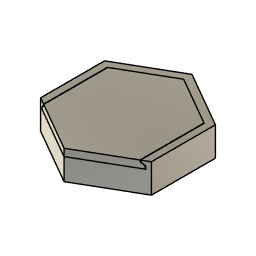
HexStore2 (Autodesk Fusion 360 design; units mm, degrees)
Autodesk Fusion 360 part; units mm, degrees
sketch "Sketch1" plane through (0, 0, 0) normal (0, 0, 1) x (1, 0, 0)
  line L0 (0, -46.188) -> (40, -23.094)
  line L1 (40, -23.094) -> (40, 23.094)
  line L2 (40, 23.094) -> (0, 46.188)
  line L3 (0, 46.188) -> (-40, 23.094)
  line L4 (-40, 23.094) -> (-40, -23.094)
  line L5 (-40, -23.094) -> (0, -46.188)
  line L6 (-46, 26.5581) -> (-46, -26.5581)
  line L7 (-46, -26.5581) -> (0, -53.1162)
  line L8 (0, -53.1162) -> (46, -26.5581)
  line L9 (46, -26.5581) -> (46, 26.5581)
  line L10 (46, 26.5581) -> (0, 53.1162)
  line L11 (0, 53.1162) -> (-46, 26.5581)
  dimension "d1" = 40
  dimension "d2" = 6
  constraint vertical L1
  measures "d1" distance of origin L5
extrude "Extrude1" add sketch "Sketch1" along normal blind 2 contours L0 L1 L2 L3 L4 L5 | L6 L7 L8 L9 L10 L11 makes body 1 in component "Case"
extrude "Extrude2" add sketch "Sketch1" along normal blind 24 bodies 1 in component "Case"
ref_plane "WorkPlane1" through (-46, -26.5581, 0) normal (0, -1, 0) x (1, 0, 0)
sketch "Sketch2" plane through (0, -26.5581, 0) normal (0, -1, 0) x (-1, 0, 0)
  line L0 (0, -24) -> (40, -24)
  line L1 (40, -24) -> (0, -24)
  line L2 (0, -24) -> (-40, -24)
  line L3 (-40, -24) -> (0, -24)
  line L4 (0, -24) -> (46, -24)
  line L5 (46, -24) -> (0, -24)
  line L6 (0, -24) -> (-46, -24)
  line L7 (-46, -24) -> (0, -24)
  line L8 (46, -24) -> (43, -24)
  line L9 (43, -24) -> (43, -18)
  line L10 (43, -18) -> (46, -18)
  line L11 (46, -18) -> (46, -24)
  line L12 (43, -24) -> (40, -24)
  line L13 (40, -24) -> (40, -18)
  line L14 (40, -18) -> (43, -18)
  line L15 (43, -18) -> (43, -24)
  line L16 (40.19, -24) -> (40.19, -23)
  line L17 (40.19, -23) -> (43, -20.19)
  line L18 (42.81, -18) -> (42.81, -20.1113)
  line L19 (42.81, -20.1113) -> (40, -22.9213)
  line L20 (0, 0) -> (0, -24)
  line L21 (-43, -24) -> (-40, -24)
  line L22 (-40, -18) -> (-43, -18)
  line L23 (-43, -18) -> (-43, -24)
  line L24 (-40, -24) -> (-40, -18)
  line L25 (-43, -24) -> (-43, -18)
  line L26 (-46, -18) -> (-46, -24)
  line L27 (-46, -24) -> (-43, -24)
  line L28 (-43, -18) -> (-46, -18)
  line L29 (-42.81, -18) -> (-42.81, -20.1113)
  line L30 (-42.81, -20.1113) -> (-40, -22.9213)
  line L31 (-40.19, -23) -> (-43, -20.19)
  line L32 (-40.19, -24) -> (-40.19, -23)
  line L33 (40, -18) -> (-40, -18)
  dimension "d7" = 3
  dimension "d8" = 6
  dimension "d9" = 3
  dimension "d10" = 6
  dimension "d11" = 45
  dimension "d12" = 0.19
  dimension "d13" = 0.19
  dimension "d14" = 0.19
  dimension "d15" = 1
  constraint horizontal L8
  constraint vertical L9
  constraint horizontal L10
  constraint vertical L11
  constraint coincident L4.end L5.start
  constraint horizontal L12
  constraint vertical L13
  constraint horizontal L14
  constraint vertical L15
  constraint coincident L12 L16.start
  constraint perpendicular L4 L16
  constraint coincident L15 L17.end
  constraint coincident L14 L18.start
  constraint perpendicular L14 L18
  constraint coincident L13 L19.end
  constraint parallel L17 L19
  constraint symmetric L4.end L20 L6.end
  constraint symmetric L8.end L20 L21.start
  constraint symmetric L9.end L20 L22.end
  constraint symmetric L10.end L20 L26.start
  constraint symmetric L0.end L20 L2.end
  constraint symmetric L13.end L20 L22.start
  constraint symmetric L16.start L20 L32.start
  constraint symmetric L16.end L20 L31.start
  constraint symmetric L17.end L20 L31.end
  constraint symmetric L18.start L20 L29.start
  constraint symmetric L18.end L20 L29.end
  constraint symmetric L19.end L20 L30.end
  measures "d7" distance of L4.end L8.end
  measures "d8" distance of L4.end L10.end
  measures "d9" distance of L8.end L0.end
  measures "d10" distance of L8.end L9.end
  measures "d11" angle of L9 L17
  measures "d12" distance of L15 L18
  measures "d13" distance of L17 L19
  measures "d14" distance of L13 L16
  measures "d15" distance of L16.start L16.end
extrude "Extrude3" cut sketch "Sketch2" along normal up to surface (-49.6521 mm away) and the other way up to surface (-26.5581 mm away) contours L0 L1 L4 L5 L13 L20 L33 | L2 L3 L6 L7 L20 L24 L33 | L4 L5 L9 L12 L13 L14 L15 L16 L17 L18 L19 | L6 L7 L21 L22 L23 L24 L25 L29 L30 L31 L32 | L13 L14 L18 L19 | L22 L24 L29 L30 bodies 1 in component "Case"
extrude "Extrude1'" add sketch "Sketch1" along normal blind 6 from surface at 18 separate body contours L0 L1 L2 L3 L4 L5 | L6 L7 L8 L9 L10 L11 makes body 2 in component "Lid"
extrude "Extrude2'" cut sketch "Sketch2" along normal up to surface (-79.6743 mm away) and the other way up to surface (-26.5581 mm away) contours L4 L5 L9 L12 L13 L14 L15 L16 L17 L18 L19 | L6 L7 L21 L22 L23 L24 L25 L29 L30 L31 L32 | L4 L5 L9 L12 L15 L16 L17 | L6 L7 L21 L23 L25 L31 L32 | L4 L5 L8 L9 L10 L11 L15 | L6 L7 L23 L25 L26 L27 L28 bodies 2 in component "Lid"
sketch "Sketch1 (2)" plane through (0, 0, 24) normal (0, 0, 1) x (-1, 0, 0) in component "Lid"
  line L0 (-40, 30.0222) -> (-40, -30.0222)
  line L1 (-40, -30.0222) -> (0, -53.1162)
  line L2 (0, -53.1162) -> (40, -30.0222)
  line L3 (40, -30.0222) -> (40, 30.0222)
  line L4 (40, 30.0222) -> (0, 53.1162)
  line L5 (0, 53.1162) -> (-40, 30.0222)
  line L6 (40, -23.094) -> (-40, -23.094)
  line L7 (-40.19, -23.094) -> (-40.19, 29.9125)
  line L8 (-40.19, 29.9125) -> (-46, 26.5581)
  line L9 (-46, 26.5581) -> (-46, -26.5581)
  line L10 (-46, -26.5581) -> (0, -53.1162)
  line L11 (0, -53.1162) -> (46, -26.5581)
  line L12 (46, -26.5581) -> (46, 26.5581)
  line L13 (46, 26.5581) -> (40.19, 29.9125)
  line L14 (40.19, 29.9125) -> (40.19, -23.094)
  line L15 (40.19, -23.094) -> (40, -23.094)
  line L16 (40, -23.094) -> (0, -46.188)
  line L17 (0, -46.188) -> (-40, -23.094)
  line L18 (-40, -23.094) -> (-40.19, -23.094)
  line L19 (-40.19, -23.094) -> (-46, -23.094)
  line L20 (40, -23.094) -> (46, -23.094)
  point P0 (40, -23.094)
  point P1 (-40, -23.094)
  constraint coincident P0 L6.start
  constraint coincident P1 L6.end
  constraint coincident L7.start L18.end
  constraint coincident L9 L19.end
  constraint perpendicular L9 L19
  constraint coincident L12 L20.end
  constraint perpendicular L12 L20
extrude "Extrude3'" cut sketch "Sketch1 (2)" against normal blind 6 contours L0 L1 L2 L3 L10 L11 L16 L17 | L0 L9 L10 L18 L19 | L3 L11 L12 L15 L20 bodies 2 in component "Lid"
sketch "Sketch1 (3)" plane through (0, 0, 18) normal (0, 0, 1) x (-1, 0, 0) in component "Case"
  line L0 (0, 53.1162) -> (-43, 28.2902)
  line L1 (-43, 28.2902) -> (-43, -23.094)
  line L2 (-43, -23.094) -> (-40, -23.094)
  line L3 (-40, -23.094) -> (-40, 23.094)
  line L4 (-40, 23.094) -> (0, 46.188)
  line L5 (0, 46.188) -> (40, 23.094)
  line L6 (40, 23.094) -> (40, -23.094)
  line L7 (40, -23.094) -> (43, -23.094)
  line L8 (43, -23.094) -> (43, 28.2902)
  line L9 (43, 28.2902) -> (0, 53.1162)
  circle A0 centre (-43, -17.094) radius 0.6
  circle A1 centre (43, -17.094) radius 0.6
  dimension "d30" = 1.2
  dimension "d31" = 1.2
  dimension "d32" = 6
  dimension "d33" = 6
  constraint coincident L1 A0.centre
  constraint coincident L8 A1.centre
  measures "d30" diameter of A0
  measures "d31" diameter of A1
  measures "d32" distance of L7.end A1.centre
  measures "d33" distance of L1.end A0.centre
extrude "Extrude4" add sketch "Sketch1 (3)" along normal blind 6 contours L1 A0 | L8 A1 picked at (-42.8071, -16.9197) picked at (42.805, -17.1385) bodies 1 in component "Case"
sketch "Sketch2 (2)" plane through (0, 0, 18) normal (0, 0, -1) x (1, 0, 0) in component "Lid"
  line L0 (40, -23.094) -> (42.81, -23.094)
  line L1 (42.81, -23.094) -> (42.81, 28.3999)
  line L2 (42.81, 28.3999) -> (0, 53.1162)
  line L3 (0, 53.1162) -> (-42.81, 28.3999)
  line L4 (-42.81, 28.3999) -> (-42.81, -23.094)
  line L5 (-42.81, -23.094) -> (-40, -23.094)
  line L6 (-40, -23.094) -> (0, -46.188)
  line L7 (0, -46.188) -> (40, -23.094)
  circle A0 centre (42.81, -17.094) radius 0.6
  circle A1 centre (-42.81, -17.094) radius 0.6
  dimension "d36" = 1.2
  dimension "d37" = 1.2
  dimension "d38" = 6
  dimension "d39" = 6
  constraint coincident L1 A0.centre
  constraint coincident L4 A1.centre
  measures "d36" diameter of A0
  measures "d37" diameter of A1
  measures "d38" distance of L0.end A0.centre
  measures "d39" distance of L4.end A1.centre
extrude "Extrude4'" cut sketch "Sketch2 (2)" against normal blind 6 contours L1 A0 | L4 A1 picked at (42.6536, -17.2187) picked at (-42.6019, -16.963) bodies 2 in component "Lid"
fillet "Fillet1" radius 1 2 edges at (42.81, 16.494, 19.0556) (42.81, 17.694, 19.0556) on bodies 2 in component "Lid"
fillet "Fillet1" radius 1 1 edges at (42.81, 23.094, 19.0556) on bodies 2 in component "Lid"
fillet "Fillet1" radius 1 1 edges at (-42.81, 23.094, 19.0556) on bodies 2 in component "Lid"
fillet "Fillet1" radius 1 2 edges at (-42.81, 16.494, 19.0556) (-42.81, 17.694, 19.0556) on bodies 2 in component "Lid"
component "Case" placed x (1, 0, 0) y (0, 1, 0) z (0, 0, 1) at (0, 0, 0)
component "Lid" placed x (1, 0, 0) y (0, 1, 0) z (0, 0, 1) at (0, 0, 0)
